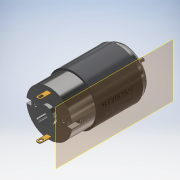
# Autodesk Inventor part: JD5B-2655W-R
Saved by Autodesk Inventor 2018 (Build 220112000, 112)
## iProperties
Created: 2018-01-11
Part Number: JD5B-2655W-R
Material: Brass, Soft Yellow
Document SubType Name: Modeling
Designer: Moochster
Density: 8.47 g/cm^3
Appearance: Semi-Polished
Mass: 30.5756 g
Surface Area: 59.0397 cm^2
Volume: 30.5756 cm^3
Author: Moochster
Autodesk Inventor part; units mm, degrees
ref_plane "XZ Plane" through (0, 0, 0) normal (0, 1, 0) x (-1, 0, 0)
ref_plane "XY Plane" through (0, 0, 0) normal (0, 0, 1) x (1, 0, 0)
sketch "Sketch1" plane through (0, 0, 0) normal (0, 0, 1) x (1, 0, 0)
  line L0 (0, 0) -> (0, 64.76)
  line L1 (0, 0) -> (1.115, 0)
  line L2 (1.115, 0) -> (1.115, 5.6)
  line L3 (1.115, 5.6) -> (5, 5.6)
  line L4 (5, 5.6) -> (5, 7.7)
  line L5 (5, 7.7) -> (13.77, 7.7)
  line L6 (13.77, 7.7) -> (13.77, 54.2)
  line L7 (13.77, 54.2) -> (5, 54.2)
  line L8 (5, 54.2) -> (5, 56.56)
  line L9 (5, 56.56) -> (1.115, 56.56)
  line L10 (1.115, 56.56) -> (1.115, 64.76)
  line L11 (1.115, 64.76) -> (0, 64.76)
  line L12 (13.77, 49.7) -> (14.865, 49.7)
  line L13 (14.865, 49.7) -> (14.865, 22.2)
  line L14 (14.865, 22.2) -> (13.77, 22.2)
  dimension "d0" = 2.23
  dimension "d1" = 5.6
  dimension "d2" = 8.2
  dimension "d3" = 2.36
  dimension "d4" = 2.1
  dimension "d5" = 10
  dimension "d6" = 10
  dimension "d7" = 46.5
  dimension "d8" = 27.54
  dimension "d9" = 14.5
  dimension "d10" = 27.5
  dimension "d11" = 29.73
  constraints: 30 end point, 11 perpendicular, 3 horizontal, 2 point on line, 1 vertical, 1 vertical alignment
  measures "d0" diameter of L2 L0
  measures "d1" distance of L1.end L2.end
  measures "d2" distance of L9.end L10.end
  measures "d3" distance of L7.end L8.end
  measures "d4" distance of L3.end L4.end
  measures "d5" diameter of L8 L0
  measures "d6" diameter of L4 L0
  measures "d7" distance of L5.end L6.end
  measures "d8" diameter of L6 L0
  measures "d9" distance from line of L5.end L14
  measures "d10" distance of L12.end L13.end
  measures "d11" diameter of L13 L0
revolve "Revolution1" add sketch "Sketch1" angle 360 about axis through (0, 0, 0) along (0, 1, 0) contours L0 L11 L10 L9 L8 L7 L6 L5 L4 L3 L2 L1
revolve "Revolution2" add sketch "Sketch1" angle 345 mid plane about axis through (0, 0, 0) along (0, 1, 0) contours L6 L12 L13 L14
fillet "Fillet1" radius 2 1 edges at (-13.77, 54.2, 0)
fillet "Fillet2" radius 0.5 2 edges at (-1.115, 0, 0) (-1.115, 64.76, 0)
sketch "Sketch2" plane through (0, 54.2, 0) normal (0, 1, 0) x (1, 0, 0)
  point P0 (0, 0)
  point P1 (-10.5, 0)
  point P2 (0, 8)
  point P3 (0, -8)
  dimension "d16" = 10.5
  dimension "d17" = 8
  dimension "d18" = 8
  constraints: 2 vertical alignment, 1 horizontal alignment
  measures "d16" distance of point (-10.5, 0) point (0, 0)
  measures "d17" distance of point (0, 0) point (0, 8)
  measures "d18" distance of point (0, -8) point (0, 0)
hole "Hole1" at (0, 54.2, -8) at (0, 54.2, 8) direction (0, -1, 0) diameter 2 depth 8 tip angle 118
sketch "Sketch3" plane through (0, 7.7, 0) normal (0, -1, 0) x (1, 0, 0)
  line L0 (1.4, 11.1) -> (-1.4, 11.1)
  line L1 (-1.4, 11.1) -> (-1.4, 11.5)
  line L2 (-1.4, 11.5) -> (1.4, 11.5)
  line L3 (1.4, 11.5) -> (1.4, 11.1)
  line L4 (1.4, -11.5) -> (-1.4, -11.5)
  line L5 (-1.4, -11.5) -> (-1.4, -11.9)
  line L6 (-1.4, -11.9) -> (1.4, -11.9)
  line L7 (1.4, -11.9) -> (1.4, -11.5)
  point P0 (0, 0)
  point P1 (0, 11.5)
  dimension "d26" = 0.4
  dimension "d27" = 2.8
  dimension "d28" = 11.5
  dimension "d29" = 11.5
  dimension "d30" = 0.4
  constraints: 16 end point, 4 parallel, 3 vertical alignment, 2 horizontal, 2 perpendicular, 1 midpoint
  measures "d26" distance of L6.end L4.start
  measures "d27" distance of L5.end L6.end
  measures "d28" distance from line of L4 point (0, 0)
  measures "d29" distance from line of L2 point (0, 0)
  measures "d30" distance of L2.end L0.start
extrude "Extrusion1" add sketch "Sketch3" along normal blind 7 separate body
fillet "Fillet3" radius 1 4 edges at (-1.4, 0.7, -11.7) (1.4, 0.7, -11.7) (-1.4, 0.7, 11.3) (1.4, 0.7, 11.3)
sketch "Sketch4" plane through (1.4, 7.7, -11.9) normal (0, 0, -1) x (-1, 0, 0)
  line L0 (1.4, -5.5) -> (1.4, -4.5) construction
  line L1 (2.15, -5.5) -> (2.15, -4.5)
  line L2 (0.65, -4.5) -> (0.65, -5.5)
  arc A0 (0.65, -5.5) -> (2.15, -5.5) centre (1.4, -5.5) ccw
  arc A1 (2.15, -4.5) -> (0.65, -4.5) centre (1.4, -4.5) ccw
  line L3 (1.8, -7) -> (1, -7) projected
  point P0 (1.4, -7.7)
  point P1 (1.4, -5)
  point P2 (1.4, -7)
  dimension "d34" = 1
  dimension "d35" = 1.5
  dimension "d36" = 2
  constraints: 8 end point, 4 point on circle, 4 tangent, 2 centre point, 2 midpoint, 1 parallel, 1 vertical, 1 vertical alignment
  measures "d34" distance of L0.start L0.end
  measures "d35" distance between parallel lines of L1 L2
  measures "d36" distance from line of L3 point (1.4, -5)
extrude "Extrusion2" cut sketch "Sketch4" against normal through all bodies 2
sketch "Sketch5" plane through (0, 7.7, 0) normal (0, -1, 0) x (1, 0, 0)
  circle A0 centre (0, 0) radius 13.77 projected
  line L0 (-13.6902, -1.48) -> (-10.7302, -1.48)
  line L1 (-10.7302, -1.48) -> (-10.7302, 1.48)
  line L2 (-10.7302, 1.48) -> (-13.6902, 1.48)
  arc A1 (-13.6522, -1.7973) -> (-13.6522, 1.7973) centre (0, 0) ccw projected
  line L3 (13.6902, -1.48) -> (10.7302, -1.48)
  line L4 (10.7302, -1.48) -> (10.7302, 1.48)
  line L5 (10.7302, 1.48) -> (13.6902, 1.48)
  point P0 (-10.7302, 0)
  dimension "d39" = 2.96
  dimension "d40" = 2.96
  constraints: 12 end point, 4 point on circle, 3 horizontal, 3 horizontal alignment, 3 perpendicular, 1 collinear, 1 midpoint
  measures "d39" distance of L0.end L1.end
  measures "d40" distance of L1.end L2.end
extrude "Extrusion3" cut sketch "Sketch5" against normal blind 5 contours A0 L3 L4 L5 | L2 L1 L0 A0 bodies 1
fillet "Fillet4" radius 2 3 edges at (-13.77, 12.7, 0) (13.75, 12.7, 0.7411) (13.75, 12.7, -0.7411)
ref_plane "Work Plane1" through (14.865, 35.95, 0) normal (1, 0, 0) x (0, 1, 0)
sketch "Sketch6" plane through (14.865, 35.95, 0) normal (1, 0, 0) x (0, 1, 0)
  line L0 (8.5587, -4.5357) -> (-12.1643, -4.5357) construction
  line L1 (-12.1643, -4.5357) -> (-12.1643, 4.5357) construction
  line L2 (-12.1643, 4.5357) -> (8.5587, 4.5357) construction
  line L3 (8.5587, 4.5357) -> (8.5587, -4.5357) construction
  line L4 (-13.75, -14.865) -> (-13.75, 14.865) projected
  point P0 (-35.95, 0)
  point P1 (-12.1643, 0)
  point P2 (-13.75, 0)
  point P3 (-13.75, 1.9403)
  point P4 (-13.75, -1.9403)
  constraints: 2 midpoint, 1 horizontal, 1 horizontal alignment, 2 other
decal "Decal1"
sketch "Sketch7" plane through (0, 7.7, 0) normal (0, -1, 0) x (1, 0, 0)
  circle A0 centre (8.465, 0) radius 0.915
  circle A1 centre (-8.465, 0) radius 0.915
  line L0 (8.465, 0) -> (-8.465, 0) construction
  point P0 (0, 0)
  point P1 (0, 0)
  dimension "d66" = 1.83
  dimension "d68" = 16.93
  constraints: 2 centre point, 2 end point, 2 horizontal alignment, 1 coincident, 1 equal radius, 1 horizontal, 1 midpoint
  measures "d66" diameter of A1
  measures "d68" distance of L0.end L0.start
extrude "Extrusion4" cut sketch "Sketch7" against normal blind 5 bodies 1
body "Solid1"
body "Solid2"
